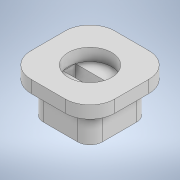
# Autodesk Inventor part: led_stand
Saved by Autodesk Inventor 2021 (Build 250183000, 183)
## iProperties
Created: 2021-03-08
Part Number: led_stand
Material: Generisch
Document SubType Name: Modeling
Designer: Tilman
Density: 1 g/cm^3
Appearance: Vorgabe
Author: Tilman
Autodesk Inventor part; units mm, degrees
ref_plane "YZ Plane" through (0, 0, 0) normal (1, 0, 0) x (0, 1, 0)
ref_plane "XZ Plane" through (0, 0, 0) normal (0, 1, 0) x (-1, 0, 0)
ref_plane "XY Plane" through (0, 0, 0) normal (0, 0, 1) x (1, 0, 0)
sketch "Skizze1" plane through (0, 0, 0) normal (0, 1, 0) x (-1, 0, 0)
  line L0 (-2, 0) -> (-7.5, 0)
  line L1 (-9.5, -2) -> (-9.5, -7.5)
  line L2 (-7.5, -9.5) -> (-2, -9.5)
  line L3 (0, -7.5) -> (0, -2)
  arc A0 (-2, -9.5) -> (0, -7.5) centre (-2, -7.5) ccw
  arc A1 (-9.5, -7.5) -> (-7.5, -9.5) centre (-7.5, -7.5) ccw
  arc A2 (-7.5, 0) -> (-9.5, -2) centre (-7.5, -2) ccw
  arc A3 (0, -2) -> (-2, 0) centre (-2, -2) ccw
  point P0 (0, 0)
  point P1 (-9.5, -9.5)
  point P2 (-9.5, 0)
  point P3 (0, -9.5)
  dimension "d0" = 9.5
  dimension "d1" = 9.5
  dimension "d2" = 2
  constraints: 8 end point, 8 point on circle, 8 point on line, 8 tangent, 4 centre point, 3 equal radius, 2 parallel, 1 horizontal, 1 perpendicular
  measures "d0" distance of point (-9.5, -9.5) point (0, -9.5)
  measures "d1" distance of point (-9.5, 0) point (-9.5, -9.5)
  measures "d2" radius of A0
extrude "Extrusion1" add sketch "Skizze1" along normal blind 5
sketch "Skizze2" plane through (0, 5, 0) normal (0, 1, 0) x (1, 0, 0)
  arc A0 (7.5, 0) -> (9.5, 2) centre (7.5, 2) ccw projected
  line L0 (9.5, 2) -> (9.5, 7.5) projected
  arc A1 (9.5, 7.5) -> (7.5, 9.5) centre (7.5, 7.5) ccw projected
  line L1 (7.5, 9.5) -> (2, 9.5) projected
  arc A2 (2, 9.5) -> (0, 7.5) centre (2, 7.5) ccw projected
  line L2 (0, 7.5) -> (0, 2) projected
  arc A3 (0, 2) -> (2, 0) centre (2, 2) ccw projected
  line L3 (2, 0) -> (7.5, 0) projected
  circle A4 centre (4.75, 4.75) radius 3.5
  line L4 (9.5, 2) -> (9.5, 7.5) projected
  arc A5 (7.5, -2) -> (11.5, 2) centre (7.5, 2) ccw
  line L5 (7.5, -2) -> (2, -2)
  arc A6 (-2, 2) -> (2, -2) centre (2, 2) ccw
  line L6 (-2, 2) -> (-2, 7.5)
  arc A7 (2, 11.5) -> (-2, 7.5) centre (2, 7.5) ccw
  line L7 (2, 11.5) -> (7.5, 11.5)
  arc A8 (11.5, 7.5) -> (7.5, 11.5) centre (7.5, 7.5) ccw
  line L8 (11.5, 7.5) -> (11.5, 2)
  point P0 (0, 0)
  point P1 (9.5, 4.75)
  point P2 (4.75, 9.5)
  dimension "d5" = 7
  dimension "d6" = 2
  constraints: 8 end point, 8 point on circle, 5 centre point, 2 midpoint, 1 horizontal alignment, 1 tangent, 1 vertical, 1 vertical alignment, 6 other
  measures "d5" diameter of A4
  measures "d6" distance between parallel lines of L1 L7
extrude "Extrusion2" add sketch "Skizze2" along normal blind 2 contours L3 A3 L2 A2 L1 A1 L0 A0 | L5 A6 L6 A7 L7 A8 L8 A5
sketch "Skizze3" plane through (4.75, 5, -4.75) normal (0, 1, 0) x (1, 0, 0)
  circle A0 centre (0, 0) radius 3.5 projected
  line L0 (-3.3541, 1) -> (3.3541, 1)
  line L1 (3.3541, 1) -> (3.3541, -1)
  line L2 (3.3541, -1) -> (-3.3541, -1)
  line L3 (-3.3541, -1) -> (-3.3541, 1)
  circle A1 centre (0, 0) radius 3.5 projected
  point P0 (-4.75, -4.75)
  dimension "d9" = 2
  constraints: 8 end point, 3 point on circle, 2 parallel, 1 horizontal, 1 perpendicular
  measures "d9" distance between parallel lines of L2 L0
extrude "Extrusion3" cut sketch "Skizze3" against normal through all contours L1 L2 L3 L0
